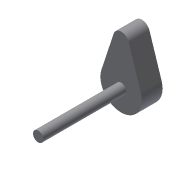
# Autodesk Inventor part: cam
Saved by Autodesk Inventor 2022 (Build 260148000, 148)
## iProperties
Created: 2004-11-26
Part Number: cam
Document SubType Name: Modeling
Designer: ndegruyther
Manufacturer: Standard
Standards Organization: Custom
Density: 1 g/cm^3
Material: Generic
Appearance: Default
Author: ndegruyther
Autodesk Inventor part; units mm, degrees
ref_plane "YZ Plane" through (0, 0, 0) normal (1, 0, 0) x (0, 1, 0)
ref_plane "XZ Plane" through (0, 0, 0) normal (0, 1, 0) x (-1, 0, 0)
ref_plane "XY Plane" through (0, 0, 0) normal (0, 0, 1) x (1, 0, 0)
sketch "Sketch1" plane through (0, 0, 0) normal (0, 0, 1) x (1, 0, 0)
  arc A0 (-5.9989, 1.3197) -> (6.0793, 1.2962) centre (0.0364, -0.6546) ccw
  arc A1 (2.3687, 12.7903) -> (-2.2437, 12.7993) centre (0.0611, 12.0454) ccw
  line L0 (-2.2437, 12.7993) -> (-5.9989, 1.3197)
  line L1 (2.3687, 12.7903) -> (6.0793, 1.2962)
  dimension "d0" = 12.7
  dimension "d8" = 12.7
  constraints: 4 end point, 4 point on circle, 4 tangent, 2 centre point
  measures "d0" diameter of A0
  measures "d8" distance of A0.centre A1.centre
extrude "Extrusion1" add sketch "Sketch1" along normal blind 6.35
sketch "Sketch2" plane through (0, 0, 6.35) normal (0, 0, 1) x (1, 0, 0)
  arc A0 (-5.2619, 3.4373) -> (5.5303, 3.1215) centre (0.0364, -0.6546) ccw projected
  circle A1 centre (0.0364, -0.6546) radius 1.5875
  dimension "d4" = 3.175
  constraints: 1 centre point, 1 coincident, 1 other
  measures "d4" diameter of A1
extrude "Extrusion2" add sketch "Sketch2" along normal blind 25.4
body "Solid1"
